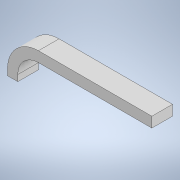
# Autodesk Inventor part: zweef-01
Saved by Autodesk Inventor 2021 (Build 250183000, 183)
## iProperties
Created: 2023-10-02
Part Number: zweef-01
Material: Generic
Document SubType Name: Modeling
Designer: Elias
Density: 1 g/cm^3
Appearance: Default
Author: Elias
Autodesk Inventor part; units mm, degrees
ref_plane "YZ Plane" through (0, 0, 0) normal (1, 0, 0) x (0, 1, 0)
ref_plane "XZ Plane" through (0, 0, 0) normal (0, 1, 0) x (-1, 0, 0)
ref_plane "XY Plane" through (0, 0, 0) normal (0, 0, 1) x (1, 0, 0)
sketch "Sketch2" plane through (0, 0, 0) normal (0, 0, 1) x (1, 0, 0)
  line L0 (0, 0) -> (5, 0)
  line L1 (5, 0) -> (5, 13)
  line L2 (0, 9.9166) -> (0, 0)
  line L3 (5, 13) -> (70, 13)
  line L4 (70, 13) -> (70, 18)
  line L5 (70, 18) -> (0, 18)
  line L6 (0, 18) -> (0, 9.9166)
  dimension "d9" = 5
  dimension "d10" = 65
  dimension "d11" = 13
  dimension "d16" = 5
  constraints: 14 end point, 4 perpendicular, 2 horizontal, 1 parallel
  measures "d9" distance of L3.end L4.end
  measures "d10" distance of L1.end L3.end
  measures "d11" distance of L0.end L1.end
  measures "d16" distance of L0.start L0.end
extrude "Extrusion2" add sketch "Sketch2" along normal blind 10
fillet "Fillet1" radius 15 1 edges at (0, 18, 5)
fillet "Fillet2" radius 10 1 edges at (5, 13, 5)
body "Solid2"
